Autodesk Inventor part; units mm, degrees
(part 2 of 2)
sketch "Sketch13" plane through (45.95, -70, 0.65) normal (1, 0, 0) x (0, 0, -1)
  line L0 (8.2783, -32.9821) -> (68.2876, -32.9821)
  line L1 (68.2876, -32.9821) -> (68.2876, -70.3608)
  line L2 (68.2876, -70.3608) -> (8.2783, -70.3608)
  line L3 (8.2783, -70.3608) -> (8.2783, -32.9821)
  line L4 (9.5497, -47.4759) -> (63.4564, -47.4759) construction
  line L5 (63.4564, -47.4759) -> (63.4564, -81.0405) construction
  line L6 (63.4564, -81.0405) -> (9.5497, -81.0405) construction
  line L7 (9.5497, -81.0405) -> (9.5497, -47.4759) construction
  line L8 (16.7977, -50.8276) -> (15.2223, -50.8276)
  line L9 (15.2223, -50.8276) -> (14.7361, -52.8438)
  line L10 (14.7361, -52.8438) -> (16.1688, -52.8438)
  line L11 (16.1688, -52.8438) -> (16.1688, -53.5699)
  line L12 (16.1688, -53.5699) -> (14.5481, -53.5699)
  line L13 (14.5481, -53.5699) -> (13.9841, -55.8325)
  line L14 (13.9841, -55.8325) -> (13.2904, -55.8325)
  line L15 (13.2904, -55.8325) -> (13.8544, -53.5699)
  line L16 (13.8544, -53.5699) -> (12.3892, -53.5699)
  line L17 (12.3892, -53.5699) -> (11.8252, -55.8325)
  line L18 (11.8252, -55.8325) -> (11.1315, -55.8325)
  line L19 (11.1315, -55.8325) -> (11.6956, -53.5699)
  line L20 (11.6956, -53.5699) -> (10.3082, -53.5699)
  line L21 (10.3082, -53.5699) -> (10.3082, -52.8438)
  line L22 (10.3082, -52.8438) -> (11.8836, -52.8438)
  line L23 (11.8836, -52.8438) -> (12.3698, -50.8276)
  line L24 (12.3698, -50.8276) -> (10.937, -50.8276)
  line L25 (10.937, -50.8276) -> (10.937, -50.1015)
  line L26 (10.937, -50.1015) -> (12.5578, -50.1015)
  line L27 (12.5578, -50.1015) -> (13.1218, -47.8325)
  line L28 (13.1218, -47.8325) -> (13.8155, -47.8325)
  line L29 (13.8155, -47.8325) -> (13.2515, -50.1015)
  line L30 (13.2515, -50.1015) -> (14.7166, -50.1015)
  line L31 (14.7166, -50.1015) -> (15.2806, -47.8325)
  line L32 (15.2806, -47.8325) -> (15.9743, -47.8325)
  line L33 (15.9743, -47.8325) -> (15.4103, -50.1015)
  line L34 (15.4103, -50.1015) -> (16.7977, -50.1015)
  line L35 (16.7977, -50.1015) -> (16.7977, -50.8276)
  line L36 (14.5481, -50.8146) -> (13.0635, -50.8146)
  line L37 (13.0635, -50.8146) -> (12.5643, -52.8568)
  line L38 (12.5643, -52.8568) -> (14.0489, -52.8568)
  line L39 (14.0489, -52.8568) -> (14.5481, -50.8146)
  line L40 (24.091, -55.8325) -> (22.8982, -55.8325)
  line L41 (22.8982, -55.8325) -> (19.3584, -48.9346)
  line L42 (19.3584, -48.9346) -> (19.3584, -55.8325)
  line L43 (19.3584, -55.8325) -> (18.3665, -55.8325)
  line L44 (18.3665, -55.8325) -> (18.3665, -47.8325)
  line L45 (18.3665, -47.8325) -> (19.8771, -47.8325)
  line L46 (19.8771, -47.8325) -> (23.0991, -54.1663)
  line L47 (23.0991, -54.1663) -> (23.0991, -47.8325)
  line L48 (23.0991, -47.8325) -> (24.091, -47.8325)
  line L49 (24.091, -47.8325) -> (24.091, -55.8325)
  spline S0 degree 2 poles (30.5675, -52.8309) (30.5675, -54.3479) (29.1088, -56.001) (27.89, -56.001) knots 0 0 0 1 2 2 2
  spline S1 degree 2 poles (27.89, -56.001) (26.6388, -56.001) (25.2061, -54.296) (25.2061, -52.8309) knots 0 0 0 1 2 2 2
  spline S2 degree 2 poles (25.2061, -52.8309) (25.2061, -51.3268) (26.6842, -49.6607) (27.89, -49.6607) knots 0 0 0 1 2 2 2
  spline S3 degree 2 poles (27.89, -49.6607) (29.1088, -49.6607) (30.5675, -51.3203) (30.5675, -52.8309) knots 0 0 0 1 2 2 2
  spline S4 degree 2 poles (29.5238, -52.8309) (29.5238, -51.6639) (28.6745, -50.5294) (27.89, -50.5294) knots 0 0 0 1 2 2 2
  spline S5 degree 2 poles (27.89, -50.5294) (27.1056, -50.5294) (26.2499, -51.6639) (26.2499, -52.8309) knots 0 0 0 1 2 2 2
  spline S6 degree 2 poles (26.2499, -52.8309) (26.2499, -53.9654) (27.1056, -55.1323) (27.89, -55.1323) knots 0 0 0 1 2 2 2
  spline S7 degree 2 poles (27.89, -55.1323) (28.668, -55.1323) (29.5238, -53.9848) (29.5238, -52.8309) knots 0 0 0 1 2 2 2
  spline S8 degree 2 poles (34.8074, -55.9751) (34.0294, -55.9751) (32.7134, -55.45) (32.2336, -54.9249) knots 0 0 0 1 2 2 2
  spline S9 degree 2 poles (32.2336, -54.9249) (31.7539, -54.4062) (31.2288, -52.8503) (31.2288, -51.839) knots 0 0 0 1 2 2 2
  spline S10 degree 2 poles (31.2288, -51.839) (31.2288, -50.8341) (31.7409, -49.343) (32.2272, -48.792) knots 0 0 0 1 2 2 2
  spline S11 degree 2 poles (32.2272, -48.792) (32.7069, -48.2539) (34.0165, -47.6898) (34.8268, -47.6898) knots 0 0 0 1 2 2 2
  spline S12 degree 2 poles (34.8268, -47.6898) (35.2288, -47.6898) (35.9354, -47.8065) (36.2336, -47.8973) knots 0 0 0 1 2 2 2
  spline S13 degree 2 poles (36.2336, -47.8973) (36.493, -47.9816) (37.0311, -48.2215) (37.2969, -48.3641) knots 0 0 0 1 2 2 2
  line L50 (37.2969, -48.3641) -> (37.2969, -49.6477)
  line L51 (37.2969, -49.6477) -> (37.2126, -49.6477)
  spline S14 degree 2 poles (37.2126, -49.6477) (37.07, -49.518) (36.6291, -49.155) (36.3114, -48.98) knots 0 0 0 1 2 2 2
  spline S15 degree 2 poles (36.3114, -48.98) (36.0067, -48.8114) (35.2871, -48.5975) (34.8204, -48.5975) knots 0 0 0 1 2 2 2
  spline S16 degree 2 poles (34.8204, -48.5975) (34.3082, -48.5975) (33.3941, -49.0189) (33.0505, -49.4208) knots 0 0 0 1 2 2 2
  spline S17 degree 2 poles (33.0505, -49.4208) (32.7134, -49.8292) (32.3374, -51.0675) (32.3374, -51.839) knots 0 0 0 1 2 2 2
  spline S18 degree 2 poles (32.3374, -51.839) (32.3374, -52.6623) (32.7328, -53.8487) (33.0764, -54.2571) knots 0 0 0 1 2 2 2
  spline S19 degree 2 poles (33.0764, -54.2571) (33.4135, -54.6526) (34.3147, -55.0545) (34.8204, -55.0545) knots 0 0 0 1 2 2 2
  spline S20 degree 2 poles (34.8204, -55.0545) (35.2806, -55.0545) (36.0651, -54.8276) (36.3698, -54.6591) knots 0 0 0 1 2 2 2
  spline S21 degree 2 poles (36.3698, -54.6591) (36.6615, -54.4905) (37.0959, -54.1404) (37.2191, -54.0172) knots 0 0 0 1 2 2 2
  line L52 (37.2191, -54.0172) -> (37.2969, -54.0172)
  line L53 (37.2969, -54.0172) -> (37.2969, -55.2879)
  spline S22 degree 2 poles (37.2969, -55.2879) (37.0311, -55.4111) (36.5643, -55.638) (36.2336, -55.7417) knots 0 0 0 1 2 2 2
  spline S23 degree 2 poles (36.2336, -55.7417) (35.8836, -55.8584) (35.2871, -55.9751) (34.8074, -55.9751) knots 0 0 0 1 2 2 2
  line L54 (42.9241, -55.8325) -> (41.9127, -55.8325)
  line L55 (41.9127, -55.8325) -> (41.9127, -52.4095)
  spline S24 degree 2 poles (41.9127, -52.4095) (41.9127, -51.9945) (41.8349, -51.2814) (41.7182, -51.0675) knots 0 0 0 1 2 2 2
  spline S25 degree 2 poles (41.7182, -51.0675) (41.5951, -50.8406) (41.1542, -50.6202) (40.7782, -50.6202) knots 0 0 0 1 2 2 2
  spline S26 degree 2 poles (40.7782, -50.6202) (40.4022, -50.6202) (39.6048, -51.0221) (39.2223, -51.3463) knots 0 0 0 1 2 2 2
  line L56 (39.2223, -51.3463) -> (39.2223, -55.8325)
  line L57 (39.2223, -55.8325) -> (38.211, -55.8325)
  line L58 (38.211, -55.8325) -> (38.211, -47.4759)
  line L59 (38.211, -47.4759) -> (39.2223, -47.4759)
  line L60 (39.2223, -47.4759) -> (39.2223, -50.497)
  spline S27 degree 2 poles (39.2223, -50.497) (39.6761, -50.0886) (40.5513, -49.6607) (41.044, -49.6607) knots 0 0 0 1 2 2 2
  spline S28 degree 2 poles (41.044, -49.6607) (41.9257, -49.6607) (42.9241, -50.8276) (42.9241, -51.9362) knots 0 0 0 1 2 2 2
  line L61 (42.9241, -51.9362) -> (42.9241, -55.8325)
  spline S29 degree 2 poles (47.6891, -55.1971) (47.5659, -55.2879) (47.151, -55.6121) (46.9565, -55.7093) knots 0 0 0 1 2 2 2
  spline S30 degree 2 poles (46.9565, -55.7093) (46.6907, -55.8519) (46.1915, -56.001) (45.7377, -56.001) knots 0 0 0 1 2 2 2
  spline S31 degree 2 poles (45.7377, -56.001) (45.3682, -56.001) (44.7004, -55.7223) (44.4476, -55.4694) knots 0 0 0 1 2 2 2
  spline S32 degree 2 poles (44.4476, -55.4694) (44.2077, -55.2231) (43.916, -54.497) (43.916, -54.095) knots 0 0 0 1 2 2 2
  spline S33 degree 2 poles (43.916, -54.095) (43.916, -53.4727) (44.4411, -52.591) (45.0116, -52.3381) knots 0 0 0 1 2 2 2
  spline S34 degree 2 poles (45.0116, -52.3381) (45.5173, -52.1048) (46.8917, -51.9297) (47.6891, -51.8843) knots 0 0 0 1 2 2 2
  line L62 (47.6891, -51.8843) -> (47.6891, -51.6898)
  spline S35 degree 2 poles (47.6891, -51.6898) (47.6891, -51.3398) (47.4751, -50.9054) (47.2806, -50.7822) knots 0 0 0 1 2 2 2
  spline S36 degree 2 poles (47.2806, -50.7822) (47.0862, -50.6591) (46.5286, -50.5813) (46.2304, -50.5813) knots 0 0 0 1 2 2 2
  spline S37 degree 2 poles (46.2304, -50.5813) (45.8803, -50.5813) (44.9338, -50.7887) (44.4606, -50.9897) knots 0 0 0 1 2 2 2
  line L63 (44.4606, -50.9897) -> (44.4022, -50.9897)
  line L64 (44.4022, -50.9897) -> (44.4022, -49.9589)
  spline S38 degree 2 poles (44.4022, -49.9589) (44.681, -49.8811) (45.7247, -49.6866) (46.2369, -49.6866) knots 0 0 0 1 2 2 2
  spline S39 degree 2 poles (46.2369, -49.6866) (46.8593, -49.6866) (47.7085, -49.8811) (48.0456, -50.1339) knots 0 0 0 1 2 2 2
  spline S40 degree 2 poles (48.0456, -50.1339) (48.3763, -50.3803) (48.7004, -51.1647) (48.7004, -51.7287) knots 0 0 0 1 2 2 2
  line L65 (48.7004, -51.7287) -> (48.7004, -55.8325)
  line L66 (48.7004, -55.8325) -> (47.6891, -55.8325)
  line L67 (47.6891, -55.8325) -> (47.6891, -55.1971)
  line L68 (47.6891, -54.3544) -> (47.6891, -52.6882)
  spline S41 degree 2 poles (47.6891, -52.6882) (47.326, -52.7206) (46.2304, -52.8309) (45.8868, -52.9346) knots 0 0 0 1 2 2 2
  spline S42 degree 2 poles (45.8868, -52.9346) (45.4849, -53.0578) (44.9597, -53.5699) (44.9597, -54.0237) knots 0 0 0 1 2 2 2
  spline S43 degree 2 poles (44.9597, -54.0237) (44.9597, -54.5424) (45.5432, -55.0675) (46.1007, -55.0675) knots 0 0 0 1 2 2 2
  spline S44 degree 2 poles (46.1007, -55.0675) (46.574, -55.0675) (47.352, -54.6591) (47.6891, -54.3544) knots 0 0 0 1 2 2 2
  line L69 (54.8333, -55.8325) -> (53.822, -55.8325)
  line L70 (53.822, -55.8325) -> (53.822, -52.4095)
  spline S45 degree 2 poles (53.822, -52.4095) (53.822, -51.9945) (53.7442, -51.2814) (53.6275, -51.0675) knots 0 0 0 1 2 2 2
  spline S46 degree 2 poles (53.6275, -51.0675) (53.5043, -50.8406) (53.0635, -50.6202) (52.6875, -50.6202) knots 0 0 0 1 2 2 2
  spline S47 degree 2 poles (52.6875, -50.6202) (52.3114, -50.6202) (51.514, -51.0221) (51.1315, -51.3463) knots 0 0 0 1 2 2 2
  line L71 (51.1315, -51.3463) -> (51.1315, -55.8325)
  line L72 (51.1315, -55.8325) -> (50.1202, -55.8325)
  line L73 (50.1202, -55.8325) -> (50.1202, -49.8292)
  line L74 (50.1202, -49.8292) -> (51.1315, -49.8292)
  line L75 (51.1315, -49.8292) -> (51.1315, -50.497)
  spline S48 degree 2 poles (51.1315, -50.497) (51.5853, -50.0886) (52.4606, -49.6607) (52.9533, -49.6607) knots 0 0 0 1 2 2 2
  spline S49 degree 2 poles (52.9533, -49.6607) (53.8349, -49.6607) (54.8333, -50.8276) (54.8333, -51.9362) knots 0 0 0 1 2 2 2
  line L76 (54.8333, -51.9362) -> (54.8333, -55.8325)
  spline S50 degree 2 poles (58.6388, -55.9686) (58.0165, -55.9686) (56.9857, -55.5861) (56.6161, -55.1971) knots 0 0 0 1 2 2 2
  spline S51 degree 2 poles (56.6161, -55.1971) (56.2466, -54.8146) (55.8382, -53.6347) (55.8382, -52.8438) knots 0 0 0 1 2 2 2
  spline S52 degree 2 poles (55.8382, -52.8438) (55.8382, -52.0529) (56.2596, -50.8989) (56.6161, -50.5099) knots 0 0 0 1 2 2 2
  spline S53 degree 2 poles (56.6161, -50.5099) (56.9727, -50.1145) (58.0294, -49.6931) (58.6388, -49.6931) knots 0 0 0 1 2 2 2
  spline S54 degree 2 poles (58.6388, -49.6931) (59.1315, -49.6931) (60.0521, -49.9719) (60.4087, -50.1534) knots 0 0 0 1 2 2 2
  line L77 (60.4087, -50.1534) -> (60.4087, -51.2879)
  line L78 (60.4087, -51.2879) -> (60.3503, -51.2879)
  spline S55 degree 2 poles (60.3503, -51.2879) (60.2401, -51.1971) (59.903, -50.9638) (59.6631, -50.8406) knots 0 0 0 1 2 2 2
  spline S56 degree 2 poles (59.6631, -50.8406) (59.4492, -50.7369) (58.8787, -50.5748) (58.6194, -50.5748) knots 0 0 0 1 2 2 2
  spline S57 degree 2 poles (58.6194, -50.5748) (57.8349, -50.5748) (56.8819, -51.7612) (56.8819, -52.8438) knots 0 0 0 1 2 2 2
  spline S58 degree 2 poles (56.8819, -52.8438) (56.8819, -53.9005) (57.8025, -55.0869) (58.6194, -55.0869) knots 0 0 0 1 2 2 2
  spline S59 degree 2 poles (58.6194, -55.0869) (59.1121, -55.0869) (60.0067, -54.6785) (60.3503, -54.3608) knots 0 0 0 1 2 2 2
  line L79 (60.3503, -54.3608) -> (60.4087, -54.3608)
  line L80 (60.4087, -54.3608) -> (60.4087, -55.4954)
  spline S60 degree 2 poles (60.4087, -55.4954) (60.2596, -55.5667) (59.8058, -55.7676) (59.6242, -55.813) knots 0 0 0 1 2 2 2
  spline S61 degree 2 poles (59.6242, -55.813) (59.3649, -55.8908) (58.9565, -55.9686) (58.6388, -55.9686) knots 0 0 0 1 2 2 2
  spline S62 degree 2 poles (63.9354, -55.9686) (62.4962, -55.9686) (60.9144, -54.3544) (60.9144, -52.8633) knots 0 0 0 1 2 2 2
  spline S63 degree 2 poles (60.9144, -52.8633) (60.9144, -51.3981) (62.4508, -49.6607) (63.6891, -49.6607) knots 0 0 0 1 2 2 2
  spline S64 degree 2 poles (63.6891, -49.6607) (64.2466, -49.6607) (65.1088, -49.9848) (65.4265, -50.3284) knots 0 0 0 1 2 2 2
  spline S65 degree 2 poles (65.4265, -50.3284) (65.7507, -50.672) (66.0943, -51.6639) (66.0943, -52.3835) knots 0 0 0 1 2 2 2
  line L81 (66.0943, -52.3835) -> (66.0943, -52.9346)
  line L82 (66.0943, -52.9346) -> (61.9387, -52.9346)
  spline S66 degree 2 poles (61.9387, -52.9346) (61.9387, -53.9783) (62.9889, -55.0869) (63.9225, -55.0869) knots 0 0 0 1 2 2 2
  spline S67 degree 2 poles (63.9225, -55.0869) (64.2531, -55.0869) (64.8949, -54.9378) (65.1542, -54.8211) knots 0 0 0 1 2 2 2
  spline S68 degree 2 poles (65.1542, -54.8211) (65.4265, -54.6915) (65.8025, -54.4646) (65.9257, -54.3608) knots 0 0 0 1 2 2 2
  line L83 (65.9257, -54.3608) -> (65.9841, -54.3608)
  line L84 (65.9841, -54.3608) -> (65.9841, -55.4629)
  spline S69 degree 2 poles (65.9841, -55.4629) (65.809, -55.5343) (65.2774, -55.7417) (65.07, -55.8001) knots 0 0 0 1 2 2 2
  spline S70 degree 2 poles (65.07, -55.8001) (64.7782, -55.8843) (64.2985, -55.9686) (63.9354, -55.9686) knots 0 0 0 1 2 2 2
  spline S71 degree 2 poles (65.1088, -52.1631) (65.0959, -51.7547) (64.9273, -51.1582) (64.7653, -50.9573) knots 0 0 0 1 2 2 2
  spline S72 degree 2 poles (64.7653, -50.9573) (64.5902, -50.7304) (64.0392, -50.4905) (63.6307, -50.4905) knots 0 0 0 1 2 2 2
  spline S73 degree 2 poles (63.6307, -50.4905) (63.2288, -50.4905) (62.6648, -50.7304) (62.4314, -50.9638) knots 0 0 0 1 2 2 2
  spline S74 degree 2 poles (62.4314, -50.9638) (62.2045, -51.2036) (61.9711, -51.7806) (61.9387, -52.1631) knots 0 0 0 1 2 2 2
  line L85 (61.9387, -52.1631) -> (65.1088, -52.1631)
  point P0 (0.65, 70)
  constraints: 8 end point, 2 parallel, 1 horizontal, 1 perpendicular, 2 other
extrude "Extrusion10" add sketch "Sketch13" along normal blind 1.69 contours L8 L9 L10 L11 L12 L13 L14 L15 L16 L17 L18 L19 L20 L21 L22 L23 L24 L25 L26 L27 L28 L29 L30 L31 L32 L33 L34 L35 | L40 L41 L42 L43 L44 L45 L46 L47 L48 L49 | S0 S1 S2 S3 | S8 S9 S10 S11 S12 S13 L50 L51 S14 S15 S16 S17 S18 S19 S20 S21 L52 L53 S22 S23 | L54 L55 S24 S25 S26 L56 L57 L58 L59 L60 S27 S28 L61 | S29 S30 S31 S32 S33 S34 L62 S35 S36 S37 L63 L64 S38 S39 S40 L65 L66 L67 | L69 L70 S45 S46 S47 L71 L72 L73 L74 L75 S48 S49 L76 | S50 S51 S52 S53 S54 L77 L78 S55 S56 S57 S58 S59 L79 L80 S60 S61 | S62 S63 S64 S65 L81 L82 S66 S67 S68 L83 L84 S69 S70
sketch "Sketch14" plane through (45.95, -70, 0.65) normal (1, 0, 0) x (0, 0, -1)
  line L0 (4.8008, -33.5793) -> (70.1894, -33.5793)
  line L1 (70.1894, -33.5793) -> (70.1894, -70.2636)
  line L2 (70.1894, -70.2636) -> (4.8008, -70.2636)
  line L3 (4.8008, -70.2636) -> (4.8008, -33.5793)
  line L4 (-0.1992, 0) -> (-0.1992, -99) projected
  line L5 (75.1894, -98.8614) -> (75.1894, 54.786) projected
  point P0 (0.65, 70)
  dimension "d36" = 5
  dimension "d37" = 5
  constraints: 8 end point, 2 parallel, 1 horizontal, 1 perpendicular
  measures "d36" distance between parallel lines of L4 L3
  measures "d37" distance between parallel lines of L5 L1
extrude "Extrusion11" add sketch "Sketch14" along normal blind 1.3
sketch "Sketch15" plane through (-44.65, -68.7, -0.65) normal (0, 1, 0) x (1, 0, 0)
  line L0 (44.65, -0.65) -> (44.65, 3.8193) construction
  line L1 (0, 73.0402) -> (0, -1.4992) projected
  line L2 (-0.65, 0) -> (89.95, 0) projected
  line L3 (0, 41.1247) -> (44.65, 41.1247)
  line L4 (44.65, 41.1247) -> (44.65, 0)
  line L5 (44.65, 0) -> (0, 0)
  line L6 (0, 0) -> (0, 41.1247)
  line L7 (0, 32) -> (0, 44.2649) projected
  line L8 (43.45, 39.9247) -> (1.2, 39.9247)
  line L9 (1.2, 39.9247) -> (1.2, 1.2)
  line L10 (1.2, 1.2) -> (43.45, 1.2)
  line L11 (43.45, 1.2) -> (43.45, 39.9247)
  line L12 (3.2, 3.2) -> (3.2, 37.9247)
  line L13 (3.2, 37.9247) -> (41.45, 37.9247)
  line L14 (41.45, 37.9247) -> (41.45, 3.2)
  line L15 (41.45, 3.2) -> (3.2, 3.2)
  line L16 (4.4, 36.7247) -> (4.4, 4.4)
  line L17 (4.4, 4.4) -> (40.25, 4.4)
  line L18 (40.25, 4.4) -> (40.25, 36.7247)
  line L19 (40.25, 36.7247) -> (4.4, 36.7247)
  line L20 (89.3, 73.0402) -> (89.3, -1.4992)
  line L21 (89.95, 0) -> (-0.65, 0)
  line L22 (89.3, 41.1247) -> (44.65, 41.1247)
  line L23 (44.65, 0) -> (89.3, 0)
  line L24 (89.3, 0) -> (89.3, 41.1247)
  line L25 (45.85, 39.9247) -> (88.1, 39.9247)
  line L26 (88.1, 39.9247) -> (88.1, 1.2)
  line L27 (88.1, 1.2) -> (45.85, 1.2)
  line L28 (45.85, 1.2) -> (45.85, 39.9247)
  line L29 (86.1, 3.2) -> (86.1, 37.9247)
  line L30 (86.1, 37.9247) -> (47.85, 37.9247)
  line L31 (47.85, 37.9247) -> (47.85, 3.2)
  line L32 (47.85, 3.2) -> (86.1, 3.2)
  line L33 (84.9, 36.7247) -> (84.9, 4.4)
  line L34 (84.9, 4.4) -> (49.05, 4.4)
  line L35 (49.05, 4.4) -> (49.05, 36.7247)
  line L36 (49.05, 36.7247) -> (84.9, 36.7247)
  dimension "d40" = 1.2
  dimension "d41" = 2
  dimension "d42" = 1.2
  constraints: 68 end point, 18 symmetric about line, 8 parallel, 4 perpendicular, 4 point on line, 1 horizontal, 1 midpoint, 1 vertical, 9 other
  measures "d40" distance between parallel lines of L3 L8
  measures "d41" distance between parallel lines of L9 L12
  measures "d42" distance between parallel lines of L12 L16
extrude "Extrusion12" [suppressed]
sketch "Sketch16" plane through (-44.65, -70, 0.65) normal (0, -1, 0) x (1, 0, 0)
  line L0 (4.337, -37.7986) -> (40.0967, -37.7986)
  line L1 (40.0967, -37.7986) -> (40.0967, -5.7136)
  line L2 (40.0967, -5.7136) -> (4.337, -5.7136)
  line L3 (4.337, -5.7136) -> (4.337, -37.7986)
  line L4 (44.65, -0.65) -> (44.65, -7.5231)
  line L5 (84.963, -37.7986) -> (49.2033, -37.7986)
  line L6 (49.2033, -37.7986) -> (49.2033, -5.7136)
  line L7 (49.2033, -5.7136) -> (84.963, -5.7136)
  line L8 (84.963, -5.7136) -> (84.963, -37.7986)
  constraints: 18 end point, 4 symmetric about line, 3 perpendicular, 1 horizontal, 1 vertical
extrude "Extrusion13" [suppressed]
ref_plane "Work Plane1" through (0, -30, 0) normal (0, 1, 0) x (-1, 0, 0)
sketch "Sketch17" plane through (0, -30, 0) normal (0, 1, 0) x (-1, 0, 0)
  line L0 (-44.65, -0.65) -> (44.65, -0.65) projected
  line L1 (-44.65, -41.7747) -> (-44.65, -0.65) projected
  line L2 (-44.65, -41.7747) -> (44.65, -41.7747) projected
  line L3 (44.65, -0.65) -> (44.65, -41.7747) projected
  line L4 (-43.45, -1.85) -> (-1.2, -1.85) projected
  line L5 (-1.2, -1.85) -> (-1.2, -40.5747) projected
  line L6 (-1.2, -40.5747) -> (-43.45, -40.5747) projected
  line L7 (-43.45, -40.5747) -> (-43.45, -1.85) projected
  line L8 (1.2, -1.85) -> (43.45, -1.85) projected
  line L9 (43.45, -1.85) -> (43.45, -40.5747) projected
  line L10 (43.45, -40.5747) -> (1.2, -40.5747) projected
  line L11 (1.2, -40.5747) -> (1.2, -1.85) projected
  line L12 (41.45, -3.85) -> (3.2, -3.85) projected
  line L13 (3.2, -38.5747) -> (41.45, -38.5747) projected
  line L14 (41.45, -38.5747) -> (41.45, -3.85) projected
  line L15 (41.45, -3.85) -> (3.2, -3.85) projected
  line L16 (3.2, -3.85) -> (3.2, -38.5747) projected
  line L17 (40.25, -5.05) -> (40.25, -37.3747) projected
  line L18 (40.25, -37.3747) -> (4.4, -37.3747) projected
  line L19 (4.4, -37.3747) -> (4.4, -5.05) projected
  line L20 (4.4, -5.05) -> (40.25, -5.05) projected
  line L21 (44.65, -0.65) -> (44.65, -32.65) projected
  line L22 (44.65, -32.65) -> (44.65, -44.9149) projected
  line L23 (45.3, -0.65) -> (-45.3, -0.65) projected
  line L24 (-41.45, -3.85) -> (-41.45, -38.5747) projected
  line L25 (-41.45, -38.5747) -> (-3.2, -38.5747) projected
  line L26 (-3.2, -38.5747) -> (-3.2, -3.85) projected
  line L27 (-3.2, -3.85) -> (-41.45, -3.85) projected
  line L28 (-4.4, -37.3747) -> (-40.25, -37.3747) projected
  line L29 (-40.25, -37.3747) -> (-40.25, -5.05) projected
  line L30 (-40.25, -5.05) -> (-4.4, -5.05) projected
  line L31 (-4.4, -5.05) -> (-4.4, -37.3747) projected
  point P0 (0, 0)
extrude "Extrusion14" add sketch "Sketch17" along normal blind 20
ref_plane "Work Plane2" through (0, -84.5, 0) normal (0, 1, 0) x (-1, 0, 0)
sketch "Sketch18" plane through (0, -84.5, 0) normal (0, 1, 0) x (-1, 0, 0)
  line L0 (12.8867, -70.3794) -> (9.6057, -70.3794) projected
  line L1 (12.8867, -74.5035) -> (12.8867, -70.3794) projected
  line L2 (11.5867, -71.6794) -> (11.5867, -74.5035) projected
  line L3 (9.6057, -71.6794) -> (11.5867, -71.6794) projected
  line L4 (9.6057, -70.3794) -> (9.6057, -71.6794) projected
  line L5 (11.5867, -74.5035) -> (12.8867, -74.5035) projected
  line L6 (12.8867, -74.5035) -> (12.8867, -70.3794) projected
  line L7 (12.8867, -70.3794) -> (9.6057, -70.3794) projected
  line L8 (9.6057, -70.3794) -> (9.6057, -71.6794) projected
  line L9 (9.6057, -71.6794) -> (11.5867, -71.6794) projected
  line L10 (11.5867, -71.6794) -> (11.5867, -74.5035) projected
  line L11 (11.5867, -74.5035) -> (12.8867, -74.5035) projected
  line L12 (-11.5867, -74.5035) -> (-11.5867, -71.6794) projected
  line L13 (-11.5867, -71.6794) -> (-9.6057, -71.6794) projected
  line L14 (-9.6057, -71.6794) -> (-9.6057, -70.3794) projected
  line L15 (-9.6057, -70.3794) -> (-12.8867, -70.3794) projected
  line L16 (-12.8867, -70.3794) -> (-12.8867, -74.5035) projected
  line L17 (-12.8867, -74.5035) -> (-11.5867, -74.5035) projected
  point P0 (0, 0)
extrude "Extrusion15" add sketch "Sketch18" along normal mid plane 40
sketch "Sketch19" plane through (0, -30, 0) normal (0, 1, 0) x (-1, 0, 0)
  line L0 (-44.65, -73.6902) -> (-44.65, 0.8492) projected
  line L1 (44.6736, -41.7221) -> (-44.65, -41.7221)
  line L2 (-44.65, -41.7221) -> (-44.65, -0.6119)
  line L3 (-44.65, -0.6119) -> (44.6736, -0.6119)
  line L4 (44.6736, -0.6119) -> (44.6736, -41.7221)
  line L5 (-40.25, -37.3747) -> (-40.25, -5.05) projected
  line L6 (-40.25, -5.05) -> (-4.4, -5.05) projected
  line L7 (-40.25, -37.3747) -> (-4.4, -37.3747)
  line L8 (-4.4, -37.3747) -> (-4.4, -5.05)
  line L9 (-4.4, -5.05) -> (-40.25, -5.05)
  line L10 (-40.25, -5.05) -> (-40.25, -37.3747)
  line L11 (4.4, -5.05) -> (40.25, -5.05) projected
  line L12 (40.25, -37.3747) -> (4.4, -37.3747) projected
  line L13 (4.4, -5.05) -> (40.25, -5.05)
  line L14 (40.25, -5.05) -> (40.25, -37.3747)
  line L15 (40.25, -37.3747) -> (4.4, -37.3747)
  line L16 (4.4, -37.3747) -> (4.4, -5.05)
  point P0 (0, 0)
  constraints: 24 end point, 6 parallel, 3 horizontal, 3 perpendicular, 1 point on line
extrude "Extrusion16" add sketch "Sketch19" against normal blind 2
equation "\"d8\" = thikness"
equation "\"d13\" = topsize + thikness"
equation "\"d20\" = d5"
equation "\"d22\" = thikness"
equation "\"d25\" = thikness"
equation "\"d26\" = thikness"
equation "\"d27\" = 2.2 * thikness"
equation "\"d30\" = 2 * thikness"
equation "\"d34\" = 1.3 * thikness"
equation "\"d38\" = thikness"
equation "\"thikness\" = 1.3"
body "Solid1"
